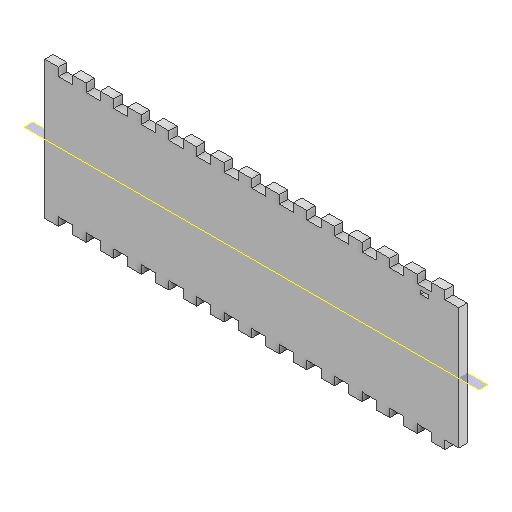
# Autodesk Inventor part: 00_Baseplate_Simmo_side4_v2
Saved by Autodesk Inventor 2022.5 (Build 265521000, 521)
## iProperties
Created: 2022-08-09
Part Number: 00_Baseplate_Simmo_side4_v2
Material: Generic
Document SubType Name: Modeling
Designer: wanghaoran
Density: 1 g/cm^3
Appearance: Default
Author: wanghaoran
Autodesk Inventor part; units mm, degrees
ref_plane "YZ Plane" through (0, 0, 0) normal (1, 0, 0) x (0, 1, 0)
ref_plane "XZ Plane" through (0, 0, 0) normal (0, 1, 0) x (-1, 0, 0)
ref_plane "XY Plane" through (0, 0, 0) normal (0, 0, 1) x (1, 0, 0)
sketch "Sketch1" plane through (0, 0, 0) normal (0, 0, 1) x (1, 0, 0)
  line L0 (-17.2654, 11) -> (-17.2654, 17) projected
  line L1 (282.6787, 11) -> (282.6787, 17) projected
  line L2 (282.6787, 17) -> (-2.7455, 17)
  line L3 (-2.7455, 17) -> (-2.7455, -83)
  line L4 (-2.7455, -83) -> (282.6787, -83)
  line L5 (282.6787, -83) -> (282.6787, 17)
  line L6 (-17.2654, 17) -> (-2.7455, 17)
  line L7 (-2.7455, 17) -> (-2.7455, -83)
  line L8 (-2.7455, -83) -> (-17.2654, -83)
  line L9 (-17.2654, -83) -> (-17.2654, 17)
  point P0 (0, 0)
  point P1 (-10, 6)
  point P2 (-10, 0)
  point P3 (-2.7455, 17)
  dimension "d0" = 100
  constraints: 16 end point, 4 parallel, 2 horizontal, 2 perpendicular
  measures "d0" distance of L3.end L2.end
extrude "Extrusion1" add sketch "Sketch1" along normal blind 6
sketch "Sketch2" plane through (0, 0, 6) normal (0, 0, 1) x (1, 0, 0)
  line L0 (282.6787, 11) -> (282.6787, 17)
  line L1 (272.7346, 17) -> (272.7346, 11) projected
  line L2 (272.7346, 11) -> (282.6787, 11)
  line L3 (262.7346, 11) -> (262.7346, 17) projected
  line L4 (252.7346, 11) -> (262.7346, 11) projected
  line L5 (252.7346, 17) -> (252.7346, 11) projected
  line L6 (272.7346, 11) -> (272.6346, 11)
  line L7 (272.6346, 11) -> (272.6346, 17)
  line L8 (272.6346, 17) -> (272.7346, 17)
  line L9 (272.7346, 17) -> (272.7346, 11)
  line L10 (282.6787, -83) -> (282.6787, 17) projected
  line L11 (282.6787, 17) -> (-17.2654, 17) projected
  line L12 (282.6787, 17) -> (272.7346, 17)
  point P0 (0, 0)
  point P1 (272.7346, 17)
  dimension "d3" = 0.1
  dimension "d4" = 6
  constraints: 14 end point, 2 parallel, 1 horizontal, 1 perpendicular
  measures "d3" distance of L7.end L8.end
  measures "d4" distance of L6.end L7.end
extrude "Extrusion2" cut sketch "Sketch2" against normal blind 6 contours L6 L7 L8 L1
sketch "Sketch3" plane through (0, 0, 6) normal (0, 0, 1) x (1, 0, 0)
  line L0 (252.7346, 17) -> (252.7346, 11) projected
  line L1 (262.7346, 11) -> (262.7346, 17) projected
  line L2 (252.7346, 17) -> (262.7346, 17) projected
  line L3 (252.7346, 17) -> (252.7346, 11) projected
  line L4 (252.7346, 11) -> (262.7346, 11) projected
  line L5 (262.7346, 11) -> (262.8346, 11)
  line L6 (262.8346, 11) -> (262.8346, 17)
  line L7 (262.8346, 17) -> (262.7346, 17)
  line L8 (262.7346, 17) -> (262.7346, 11)
  line L9 (252.7346, 11) -> (252.6346, 11)
  line L10 (252.6346, 11) -> (252.6346, 17)
  line L11 (252.6346, 17) -> (252.7346, 17)
  line L12 (252.7346, 17) -> (252.7346, 11)
  point P0 (0, 0)
  dimension "d11" = 0.1
  dimension "d12" = 6
  dimension "d13" = 0.1
  dimension "d14" = 6
  constraints: 16 end point, 4 parallel, 2 horizontal, 2 perpendicular
  measures "d11" distance of L7.end L6.end
  measures "d12" distance of L6.end L5.end
  measures "d13" distance of L10.end L11.end
  measures "d14" distance of L9.end L10.end
extrude "Extrusion3" cut sketch "Sketch3" against normal blind 6
pattern_linear "Rectangular Pattern1" count 14 spacing 20 along (-1, 0, 0) of "Extrusion3"
ref_plane "Work Plane1" through (-17.2654, -33, 0) normal (0, -1, 0) x (1, 0, 0)
mirror "Mirror1" about plane through (-17.2654, -33, 0) normal (0, -1, 0) of "Extrusion3"
pattern_linear "Rectangular Pattern2" count 14 spacing 20 along (-1, 0, 0) count 2 spacing 20 along (1, 0, 0) of "Extrusion3", "Mirror1"
sketch "Sketch4" plane through (0, 0, 6) normal (0, 0, 1) x (1, 0, 0)
  line L0 (280.4846, 6.6) -> (274.9846, 6.6)
  line L1 (274.9846, 6.6) -> (274.9846, 9)
  line L2 (274.9846, 9) -> (280.4846, 9)
  line L3 (280.4846, 9) -> (280.4846, 6.6)
  line L4 (272.6346, 11) -> (272.6346, 17) projected
  line L5 (282.6787, 17) -> (-17.2654, 17) projected
  line L6 (260.4846, 5.6) -> (254.9846, 5.6)
  line L7 (254.9846, 5.6) -> (254.9846, 8)
  line L8 (254.9846, 8) -> (260.4846, 8)
  line L9 (260.4846, 8) -> (260.4846, 5.6)
  line L10 (262.8346, 11) -> (252.6346, 11) projected
  line L11 (252.6346, 11) -> (252.6346, 17) projected
  point P0 (0, 0)
  point P1 (262.8346, 17)
  dimension "d26" = 5.5
  dimension "d27" = 2.4
  dimension "d28" = 2.35
  dimension "d29" = 8
  dimension "d32" = 5.5
  dimension "d33" = 2.4
  dimension "d34" = 3
  dimension "d35" = 2.35
  constraints: 16 end point, 4 parallel, 2 horizontal, 2 perpendicular
  measures "d26" distance of L1.end L2.end
  measures "d27" distance of L0.end L1.end
  measures "d28" distance between parallel lines of L4 L1
  measures "d29" distance between parallel lines of L2 L5
  measures "d32" distance of L7.end L8.end
  measures "d33" distance of L6.end L7.end
  measures "d34" distance between parallel lines of L10 L8
  measures "d35" distance between parallel lines of L11 L7
extrude "Extrusion4" cut sketch "Sketch4" against normal through all contours L6 L7 L8 L9
pattern_linear "Rectangular Pattern3" [suppressed]
body "Solid1"
